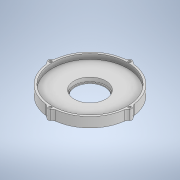
# Autodesk Inventor part: End
Saved by Autodesk Inventor 2021 (Build 250183000, 183)
## iProperties
Created: 2022-08-14
Part Number: End
Material: Ogólny
Document SubType Name: Modeling
Designer: MicnedSQ
Density: 1 g/cm^3
Appearance: Domyślna
Author: MicnedSQ
Autodesk Inventor part; units mm, degrees
ref_plane "YZ Plane" through (0, 0, 0) normal (1, 0, 0) x (0, 1, 0)
ref_plane "XZ Plane" through (0, 0, 0) normal (0, 1, 0) x (-1, 0, 0)
ref_plane "XY Plane" through (0, 0, 0) normal (0, 0, 1) x (1, 0, 0)
sketch "Szkic1" plane through (0, 0, 0) normal (0, 1, 0) x (-1, 0, 0)
  circle A0 centre (0, 0) radius 40
  circle A1 centre (0, 0) radius 15
  dimension "d0" = 80
  dimension "d1" = 30
  constraints: 2 centre point, 2 coincident
  measures "d0" diameter of A0
  measures "d1" diameter of A1
extrude "Wyciągnięcie proste1" add sketch "Szkic1" along normal blind 1
sketch "Szkic2" plane through (0, 1, 0) normal (0, 1, 0) x (1, 0, 0)
  circle A0 centre (0, 0) radius 40
  circle A1 centre (0, 0) radius 16.05
  dimension "d4" = 32.1
  constraints: 2 centre point, 2 coincident
  measures "d4" diameter of A1
extrude "Wyciągnięcie proste2" add sketch "Szkic2" along normal blind 4
sketch "Szkic3" plane through (0, 5, 0) normal (0, 1, 0) x (1, 0, 0)
  circle A0 centre (0, 0) radius 40
  circle A1 centre (0, 0) radius 38
  dimension "d7" = 76
  constraints: 2 centre point, 2 coincident
  measures "d7" diameter of A1
extrude "Wyciągnięcie proste3" add sketch "Szkic3" along normal blind 5
sketch "Szkic4" plane through (0, 0, 0) normal (0, -1, 0) x (1, 0, 0)
  circle A0 centre (0, 0) radius 40 projected
  circle A1 centre (0, 40) radius 1.35
  circle A2 centre (0, 40) radius 2.5
  point P0 (2.4988, 39.9219)
  point P1 (-2.4988, 39.9219)
  dimension "d10" = 2.7
  dimension "d11" = 5
  constraints: 2 centre point, 1 coincident, 2 other
  measures "d10" diameter of A1
  measures "d11" diameter of A2
extrude "Wyciągnięcie proste4" add sketch "Szkic4" against normal blind 10 contours A0 A1 A2 | A0 A1 picked at (1.9426, 40.8023) picked at (0.0508, 40.4454)
fillet "Zaokrąglenie1" radius 5 4 edges at (2.4988, 0.5, 39.9219) (2.4988, 5.5, 39.9219) (-2.4988, 5.5, 39.9219) (-2.4988, 0.5, 39.9219)
sketch "Szkic5" plane through (0, 0, 0) normal (0, -1, 0) x (1, 0, 0)
  circle A0 centre (0, 40) radius 1.35
  point P0 (0, 0)
  dimension "d15" = 2.7
  constraints: 1 centre point
  measures "d15" diameter of A0
extrude "Wyciągnięcie proste5" cut sketch "Szkic5" against normal blind 10
sketch "Szkic6" plane through (0, 0, 0) normal (0, -1, 0) x (1, 0, 0)
  circle A0 centre (0, 40) radius 1.35 projected
  circle A1 centre (0, 40) radius 2.25
  point P0 (0, 0)
  dimension "d18" = 4.5
  constraints: 1 centre point, 1 coincident
  measures "d18" diameter of A1
extrude "Wyciągnięcie proste6" cut sketch "Szkic6" against normal blind 3
pattern_circular "Szyk kołowy1" count 4 over 360 about axis through (0, 0, 0) along (0, 1, 0) of "Wyciągnięcie proste5", "Wyciągnięcie proste6", "Zaokrąglenie1", "Wyciągnięcie proste4"
